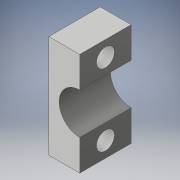
# Autodesk Inventor part: reverse gear connecting rod 1
Saved by Autodesk Inventor 2017 (Build 210142000, 142)
## iProperties
Created: 2018-10-30
Part Number: reverse gear connecting rod 1
Material: Generic
Document SubType Name: Modeling
Designer: User
Density: 1 g/cm^3
Appearance: Default
Author: User
Autodesk Inventor part; units mm, degrees
ref_plane "YZ Plane" through (0, 0, 0) normal (1, 0, 0) x (0, 1, 0)
ref_plane "XZ Plane" through (0, 0, 0) normal (0, 1, 0) x (-1, 0, 0)
ref_plane "XY Plane" through (0, 0, 0) normal (0, 0, 1) x (1, 0, 0)
sketch "Sketch1" plane through (0, 0, 0) normal (0, 1, 0) x (-1, 0, 0)
  line L0 (0, 0) -> (6, 0)
  line L1 (6, 0) -> (6, -20)
  line L2 (6, -20) -> (0, -20)
  arc A0 (0, -14) -> (0, -6) centre (0, -10) ccw
  line L3 (0, -20) -> (0, -14)
  line L4 (0, -6) -> (0, 0)
  dimension "d0" = 6
  dimension "d1" = 20
  dimension "d2" = 6
  dimension "d3" = 20
  dimension "d8" = 8
  dimension "d11" = 90
  dimension "d14" = 6
  dimension "d15" = 6
  constraints: 10 end point, 2 perpendicular, 2 point on circle, 1 centre point, 1 horizontal, 1 parallel
  measures "d0" distance of L0.start L0.end
  measures "d1" distance of L0.end L1.end
  measures "d2" distance of L1.end L2.end
  measures "d3" distance of L2.end L0.start
  measures "d8" diameter of A0
  measures "d11" angle of L3 L0
  measures "d14" distance from line of L4.start L0
  measures "d15" distance from line of A0.centre L1
extrude "Extrusion1" add sketch "Sketch1" along normal blind 10
sketch "Sketch2" plane through (0, 0, 0) normal (1, 0, 0) x (0, 0, -1)
  line L0 (20, 0) -> (14, 0) projected
  line L1 (20, 0) -> (20, 10) projected
  line L2 (14, 10) -> (20, 10) projected
  line L3 (14, 0) -> (14, 10) projected
  line L4 (6, 0) -> (0, 0) projected
  line L5 (6, 0) -> (6, 10) projected
  line L6 (0, 10) -> (6, 10) projected
  line L7 (0, 0) -> (0, 10) projected
  circle A0 centre (17, 5) radius 1.75
  circle A1 centre (3, 5) radius 1.75
  dimension "d17" = 3.5
  dimension "d18" = 3.5
  dimension "d20" = 14
  dimension "d21" = 5
  dimension "d22" = 3
  dimension "d23" = 5
  constraints: 2 centre point
  measures "d17" diameter of A0
  measures "d18" diameter of A1
  measures "d20" distance of A1.centre A0.centre
  measures "d21" distance from line of L2 A0.centre
  measures "d22" distance from line of A0.centre L1
  measures "d23" distance from line of A1.centre L0
extrude "Extrusion2" cut sketch "Sketch2" against normal through all contours A0 | A1
body "Solid1"
